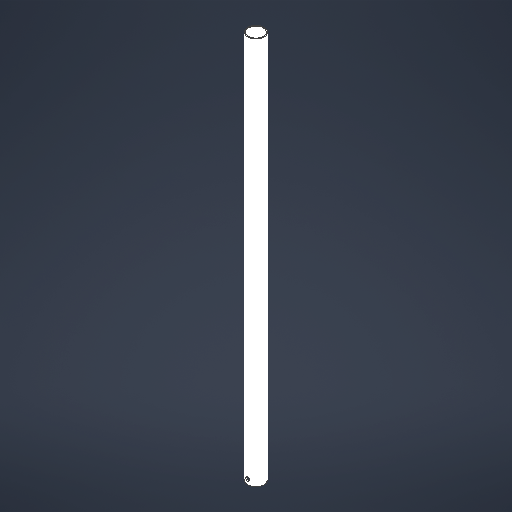
# Autodesk Inventor part: Pieza38
Saved by Autodesk Inventor 2026.2 (Build 302298000, 298)
## iProperties
Created: 2026-01-02
Part Number: Pieza38
Material: Genérico
Document SubType Name: Modeling
Designer: vicho
Density: 1 g/cm^3
Appearance: Valor por defecto
Author: vicho
Autodesk Inventor part; units mm, degrees
ref_plane "YZ Plane" through (0, 0, 0) normal (1, 0, 0) x (0, 1, 0)
ref_plane "XZ Plane" through (0, 0, 0) normal (0, 1, 0) x (-1, 0, 0)
sketch "Boceto1" plane through (0, 0, 0) normal (0, 1, 0) x (-1, 0, 0)
  circle A0 centre (0, 0) radius 17.5
  dimension "d0" = 35
  constraints: 1 centre point, 1 coincident
  measures "d0" diameter of A0
extrude "Extrusión1" add sketch "Boceto1" along normal blind 805
shell "Vaciado1" thickness 2 removed faces 2 at (-4.3663, 0, -1.0762) at (-4.3663, 805, -1.0762)
ref_plane "Plano de trabajo1" through (0, 0, 17.5) normal (0, 0, 1) x (1, 0, 0)
sketch "Boceto2" plane through (0, 0, 17.5) normal (0, 0, 1) x (1, 0, 0)
  line L0 (0, 81.1949) -> (0, -92.1127) construction
  line L1 (-146.6766, 0) -> (158.2781, 0) construction
  circle A0 centre (0, 10) radius 4
  point P0 (0, 0)
  dimension "d5" = 8
  dimension "d6" = 10
  constraints: 4 end point, 3 point on line, 1 centre point, 1 horizontal, 1 vertical
  measures "d5" diameter of A0
  measures "d6" distance from line of L1 A0.centre
extrude "Extrusión2" cut sketch "Boceto2" against normal blind 50
